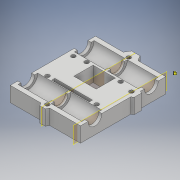
# Autodesk Inventor part: custom
Saved by Autodesk Inventor 2018 (Build 220112000, 112)
## iProperties
Created: 2017-08-29
Part Number: custom
Material: Generic
Document SubType Name: Modeling
Designer: Jasper
Density: 1 g/cm^3
Appearance: Default
Author: Jasper
Autodesk Inventor part; units mm, degrees
ref_plane "YZ Plane" through (0, 0, 0) normal (1, 0, 0) x (0, 1, 0)
ref_plane "XZ Plane" through (0, 0, 0) normal (0, 1, 0) x (-1, 0, 0)
ref_plane "XY Plane" through (0, 0, 0) normal (0, 0, 1) x (1, 0, 0)
sketch "Sketch1" plane through (0, 0, 0) normal (0, 0, 1) x (1, 0, 0)
  line L0 (-28, -34) -> (28, -34)
  line L1 (28, -34) -> (28, 34)
  line L2 (28, 34) -> (-28, 34)
  line L3 (-28, 34) -> (-28, -34)
  line L4 (-28, -34) -> (28, 34) construction
  line L5 (28, -34) -> (-28, 34) construction
  point P0 (0, 0)
  dimension "d0" = 56
  dimension "d1" = 68
  constraints: 12 end point, 2 midpoint, 2 parallel, 1 horizontal, 1 perpendicular
  measures "d0" distance of L1.end L2.end
  measures "d1" distance of L0.end L1.end
extrude "Extrusion1" add sketch "Sketch1" along normal blind 12
sketch "Sketch2" plane through (28, -34, 0) normal (1, 0, 0) x (0, 0, -1)
  line L0 (0, 34) -> (-11.654, 34)
  line L1 (-11.654, 34) -> (-11.654, 11.5)
  line L2 (-11.654, 34) -> (-11.654, 56.5)
  circle A0 centre (-11.654, 11.5) radius 5.5
  circle A1 centre (-11.654, 56.5) radius 5.5
  dimension "d4" = 22.5
  dimension "d5" = 11
  dimension "d6" = 11
  constraints: 6 end point, 2 centre point, 2 coincident, 1 horizontal, 1 perpendicular, 1 symmetric about line
  measures "d4" distance of L0.end L1.end
  measures "d5" diameter of A0
  measures "d6" diameter of A1
extrude "Extrusion2" cut sketch "Sketch2" against normal up to surface (56 mm away)
ref_plane "Work Plane1" through (25.5, -34, 0) normal (1, 0, 0) x (0, 0, -1)
sketch "Sketch3" plane through (25.5, -34, 0) normal (1, 0, 0) x (0, 0, -1)
  line L0 (-12, 51.0109) -> (-12, 16.9891) projected
  line L1 (-12, 61.9891) -> (-12, 68) projected
  line L2 (-12, 51.0109) -> (-12, 61.9891)
  line L3 (-12, 16.9891) -> (-12, 6.0109)
  circle A0 centre (-12, 11.5) radius 7.85
  circle A1 centre (-12, 56.5) radius 7.85
  point P0 (0, 34)
  dimension "d9" = 15.7
  dimension "d10" = 15.7
  constraints: 4 end point, 2 centre point, 2 midpoint, 2 vertical
  measures "d9" diameter of A0
  measures "d10" diameter of A1
extrude "Extrusion3" cut sketch "Sketch3" against normal blind 24.5
ref_plane "Work Plane2" through (0, -34, 0) normal (1, 0, 0) x (0, 0, -1)
mirror "Mirror1" about plane through (0, -34, 0) normal (1, 0, 0) of "Extrusion3"
sketch "Sketch10" plane through (0, 0, 12) normal (0, 0, 1) x (1, 0, 0)
  line L0 (-8.9, 12.925) -> (8.9, 12.925)
  line L1 (8.9, 14.65) -> (8.9, -2.375)
  line L2 (8.9, -2.375) -> (-8.9, -2.375)
  line L3 (-8.9, -2.375) -> (-8.9, 12.925)
  line L4 (10.4, -4.375) -> (-10.4, -4.375) projected
  line L5 (10.4, 10.325) -> (10.4, -4.375) projected
  line L6 (-10.4, -4.375) -> (-10.4, 10.325) projected
  line L7 (-1, 14.65) -> (-25.5, 14.65) projected
  line L8 (-28, 17.0109) -> (-28, -17.0109) projected
  line L9 (28, -17.0109) -> (28, 17.0109) projected
  line L10 (-28, 10.325) -> (28, 10.325) projected
  line L11 (25.5, 14.65) -> (1, 14.65) projected
  line L12 (-1, -15.073) -> (1, -15.073)
  line L13 (0, -15.073) -> (0, -10.325)
  line L14 (28, -10.325) -> (-28, -10.325) projected
  line L15 (-15, -13.999) -> (15, -13.999)
  line L16 (15, -13.999) -> (15, -11.399)
  line L17 (15, -11.399) -> (-15, -11.399)
  line L18 (-15, -11.399) -> (-15, -13.999)
  line L19 (-15, -13.999) -> (15, -11.399) construction
  line L20 (15, -13.999) -> (-15, -11.399) construction
  line L21 (1, -14.65) -> (25.5, -14.65) projected
  point P0 (0, 0)
  point P1 (-28, 6.925)
  point P2 (28, 4.325)
  point P3 (21.4, 10.325)
  point P4 (0, -12.699)
  dimension "d82" = 2
  dimension "d83" = 1.5
  dimension "d84" = 1.5
  dimension "d105" = 15.3
  dimension "d116" = 2.6
  dimension "d117" = 30
  dimension "d152" = 0.651
  constraints: 24 end point, 5 midpoint, 4 parallel, 3 horizontal, 2 perpendicular, 2 point on line
  measures "d82" distance between parallel lines of L4 L2
  measures "d83" distance between parallel lines of L5 L1
  measures "d84" distance between parallel lines of L6 L3
  measures "d105" distance between parallel lines of L2 L0
  measures "d116" distance of L15.end L16.end
  measures "d117" distance of L15.start L15.end
  measures "d152" distance between parallel lines of L21 L15
extrude "Extrusion9" cut sketch "Sketch10" against normal up to surface (12 mm away) contours L17 L16 L15 L13 | L13 L15 L18 L17 | L0 L1 L10 L3 | L10 L1 L2 L3
sketch "Sketch12" plane through (0, 0, 12) normal (0, 0, 1) x (1, 0, 0)
  line L0 (-28, 10.325) -> (28, 10.325) projected
  line L1 (-10.4, 10.325) -> (-8.9, 10.325)
  line L2 (-8.9, 12.925) -> (-8.9, -2.375) projected
  line L3 (-1, 14.65) -> (-25.5, 14.65) projected
  line L4 (-8.9, 14.65) -> (-8.9, 10.325)
  line L5 (-8.9, 12.4875) -> (-13.55, 12.4875) construction
  circle A0 centre (-13.55, 12.4875) radius 1.65
  line L6 (28, -17.0109) -> (28, 17.0109) construction
  line L7 (28, 5.325) -> (21.4, 5.325) construction
  line L8 (21.4, 5.325) -> (21.4, 14.65) construction
  line L9 (21.4, 14.65) -> (28, 14.65) construction
  line L10 (28, 14.65) -> (28, 5.325) construction
  line L11 (21.4, 5.825) -> (21.4, 10.325) construction
  line L12 (25.5, 14.65) -> (1, 14.65) projected
  line L13 (21.4, 14.65) -> (28, 5.325) construction
  circle A1 centre (24.7, 9.9875) radius 1.65
  line L14 (-28, -34) -> (28, -34) projected
  line L15 (0, -34) -> (0, 34)
  circle A2 centre (13.55, 12.4875) radius 1.65
  line L16 (-15, -11.399) -> (-15, -13.999) projected
  line L17 (-15, -12.699) -> (-19.65, -12.699) construction
  circle A3 centre (-19.65, -12.699) radius 1.65
  circle A4 centre (19.65, -12.699) radius 1.65
  line L18 (-28, 7.925) -> (-18, 7.925) construction
  line L19 (-18, 7.925) -> (-18, 14.65) construction
  line L20 (-18, 14.65) -> (-28, 14.65) construction
  line L21 (-28, 14.65) -> (-28, 7.925) construction
  line L22 (-18, 10.325) -> (-18, 8.425) construction
  line L23 (-28, 14.65) -> (-18, 7.925) construction
  circle A5 centre (-23, 11.2875) radius 1.65
  line L24 (-28, 30.85) -> (28, 30.85) construction
  circle A6 centre (0, 32.5) radius 1.65
  line L25 (-25.5, 30.35) -> (-1, 30.35) projected
  line L26 (28, -34) -> (28, 34) projected
  line L27 (28, 0) -> (-28, 0)
  line L28 (-28, -30.85) -> (28, -30.85) construction
  circle A7 centre (0, -32.5) radius 1.65
  point P0 (0, 0)
  dimension "d118" = 4.65
  dimension "d119" = 3.3
  dimension "d121" = 3.3
  dimension "d122" = 4.65
  dimension "d123" = 3.3
  dimension "d124" = 3.3
  dimension "d125" = 3.3
  dimension "d126" = 0.5
  constraints: 36 end point, 8 centre point, 7 horizontal, 6 midpoint, 5 symmetric about line, 4 collinear, 4 parallel, 3 perpendicular, 3 point on line, 2 coincident, 1 tangent, 1 vertical, 3 other
  measures "d118" distance of L5.start L5.end
  measures "d119" diameter of A0
  measures "d121" diameter of A1
  measures "d122" distance of L17.start L17.end
  measures "d123" diameter of A3
  measures "d124" diameter of A5
  measures "d125" diameter of A6
  measures "d126" distance between parallel lines of L25 L24
extrude "Extrusion11" cut sketch "Sketch12" against normal up to surface (12 mm away) contours A6 | A5 L0 | L0 A5 | A1 L0 | L0 A1 | A7 L14 L15 | L15 L14 A7 | L14 A7 | A0 | A2 | A3 | A4
sketch "Sketch13" plane through (0, 0, 0) normal (0, 0, -1) x (-1, 0, 0)
  line L0 (3.4064, 38.1506) -> (5.8027, 34)
  line L1 (-5.8027, 34) -> (-3.4064, 38.1506)
  line L2 (-3.4064, 38.1506) -> (3.4064, 38.1506)
  line L3 (0, 34) -> (0, 32.2506)
  line L4 (-28, 34) -> (28, 34) projected
  line L5 (-28, 34) -> (28, 34) projected
  line L6 (-5.8027, 34) -> (5.8027, 34)
  line L7 (-28, -34) -> (-28, 34) projected
  line L8 (-28, 0) -> (28, 0)
  circle A0 centre (-24.7, 9.9875) radius 1.65 projected
  line L9 (-29.7, 12.8743) -> (-24.7, 15.761)
  line L10 (-24.7, 15.761) -> (-19.7, 12.8743)
  line L11 (-19.7, 12.8743) -> (-19.7, 7.1007)
  line L12 (-19.7, 7.1007) -> (-24.7, 4.214)
  line L13 (-24.7, 4.214) -> (-29.7, 7.1007)
  line L14 (-29.7, 7.1007) -> (-29.7, 12.8743)
  line L15 (-28, 13.8557) -> (-28, 6.1193)
  circle A1 centre (0, -32.5) radius 1.65 projected
  line L16 (-2.189, -36.2915) -> (-3.512, -34)
  line L17 (3.512, -34) -> (2.189, -36.2915)
  line L18 (2.189, -36.2915) -> (-2.189, -36.2915)
  line L19 (28, -34) -> (-28, -34) projected
  line L20 (-3.512, -34) -> (3.512, -34)
  point P0 (0, 0)
  dimension "d131" = 1.7494
  dimension "d142" = 10
  constraints: 34 end point, 8 point on line, 4 coincident, 2 midpoint, 1 horizontal, 1 vertical, 21 other
  measures "d131" distance of L3.start L3.end
  measures "d142" distance between parallel lines of L11 L14
extrude "Extrusion12" add sketch "Sketch13" against normal up to surface (12 mm away) contours L19 A1 L17 L18 L16 | L7 L13 L14 L9 | L0 L4 L1 L2 | L19 A1 picked at (-0.1173, -34.0374)
sketch "Sketch14" plane through (0, 0, 0) normal (0, 0, -1) x (-1, 0, 0)
  circle A0 centre (0, 32.5) radius 1.65 projected
  line L0 (-1.65, 32.5) -> (1.65, 32.5) construction
  line L1 (1.7321, 35.5) -> (3.4641, 32.5)
  line L2 (3.4641, 32.5) -> (1.7321, 29.5)
  line L3 (1.7321, 29.5) -> (-1.7321, 29.5)
  line L4 (-1.7321, 29.5) -> (-3.4641, 32.5)
  line L5 (-3.4641, 32.5) -> (-1.7321, 35.5)
  line L6 (-1.7321, 35.5) -> (1.7321, 35.5)
  circle A1 centre (23, 11.2875) radius 1.65 projected
  line L7 (26, 9.5554) -> (23, 7.8234)
  line L8 (23, 7.8234) -> (20, 9.5554)
  line L9 (20, 9.5554) -> (20, 13.0196)
  line L10 (20, 13.0196) -> (23, 14.7516)
  line L11 (23, 14.7516) -> (26, 13.0196)
  line L12 (26, 13.0196) -> (26, 9.5554)
  circle A2 centre (-24.7, 9.9875) radius 1.65 projected
  line L13 (-27.7, 11.7196) -> (-24.7, 13.4516)
  line L14 (-24.7, 13.4516) -> (-21.7, 11.7196)
  line L15 (-21.7, 11.7196) -> (-21.7, 8.2554)
  line L16 (-21.7, 8.2554) -> (-24.7, 6.5234)
  line L17 (-24.7, 6.5234) -> (-27.7, 8.2554)
  line L18 (-27.7, 8.2554) -> (-27.7, 11.7196)
  circle A3 centre (0, -32.5) radius 1.65 projected
  line L19 (1.7321, -29.5) -> (3.4641, -32.5)
  line L20 (3.4641, -32.5) -> (1.7321, -35.5)
  line L21 (1.7321, -35.5) -> (-1.7321, -35.5)
  line L22 (-1.7321, -35.5) -> (-3.4641, -32.5)
  line L23 (-3.4641, -32.5) -> (-1.7321, -29.5)
  line L24 (-1.7321, -29.5) -> (1.7321, -29.5)
  point P0 (0, 0)
  dimension "d138" = 6
  dimension "d139" = 6
  dimension "d140" = 6
  dimension "d141" = 6
  constraints: 50 end point, 4 coincident, 2 point on circle, 1 horizontal, 52 other
  measures "d138" distance between parallel lines of L3 L6
  measures "d139" distance between parallel lines of L12 L9
  measures "d140" distance between parallel lines of L15 L18
  measures "d141" distance between parallel lines of L21 L24
extrude "Extrusion13" cut sketch "Sketch14" against normal blind 3.1
body "Solid1"
